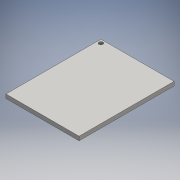
# Autodesk Inventor part: Крышка контейнера
Saved by Autodesk Inventor 2016 SP1 (Build 200210100, 210)
## iProperties
Created: 2016-05-03
Part Number: Крышка контейнера
Material: Типовые
Document SubType Name: Modeling
Designer: AS
Density: 1 g/cm^3
Appearance: По умолчанию
Author: AS
Autodesk Inventor part; units mm, degrees
ref_plane "YZ Plane" through (0, 0, 0) normal (1, 0, 0) x (0, 1, 0)
ref_plane "XZ Plane" through (0, 0, 0) normal (0, 1, 0) x (-1, 0, 0)
ref_plane "XY Plane" through (0, 0, 0) normal (0, 0, 1) x (1, 0, 0)
sketch "Эскиз1" plane through (0, 0, 0) normal (0, 0, 1) x (1, 0, 0)
  line L0 (63.5, -82.5) -> (-63.5, -82.5) projected
  line L1 (-63.5, -82.5) -> (-63.5, 82.5) projected
  line L2 (63.5, 82.5) -> (63.5, -82.5) projected
  line L3 (-63.5, 82.5) -> (63.5, 82.5) projected
  point P0 (0, 0)
extrude "Выдавливание1" add sketch "Эскиз1" along normal blind 5
sketch "Эскиз2" plane through (0, 0, 0) normal (0, 0, 1) x (1, 0, 0)
  line L0 (-63.5, -82.5) -> (-63.5, 82.5) projected
  line L1 (-63.5, 82.5) -> (63.5, 82.5) projected
  line L2 (63.5, 82.5) -> (63.5, -82.5) projected
  line L3 (63.5, -82.5) -> (-63.5, -82.5) projected
  line L4 (-61.7, 80.7) -> (-61.7, -80.7)
  line L5 (-61.7, -80.7) -> (61.7, -80.7)
  line L6 (61.7, -80.7) -> (61.7, 80.7)
  line L7 (61.7, 80.7) -> (-61.7, 80.7)
  point P0 (0, 0)
  dimension "d2" = 1.8
  constraints: 8 end point, 3 other
  measures "d2" distance between parallel lines of L0 L4
extrude "Выдавливание2" add sketch "Эскиз2" against normal blind 2
hole "Отверстие1" at (-57.302, 76.302, 5) direction (0, 0, -1) diameter 4 end through all counterbore diameter 7 counterbore depth 3
